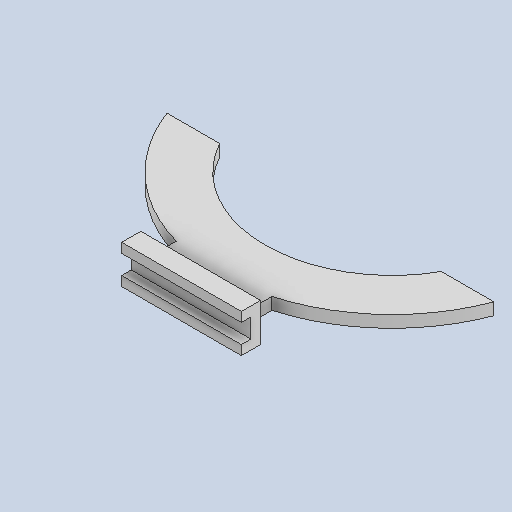
# Autodesk Inventor part: BigHolder
Saved by Autodesk Inventor 2025 (Build 290162000, 162)
## iProperties
Created: 2025-08-07
Part Number: BigHolder
Material: Generic
Document SubType Name: Modeling
Designer: Pravoslav
Density: 1 g/cm^3
Appearance: Default
Author: Pravoslav
Autodesk Inventor part; units mm, degrees
ref_plane "YZ Plane" through (0, 0, 0) normal (1, 0, 0) x (0, 1, 0)
ref_plane "XZ Plane" through (0, 0, 0) normal (0, 1, 0) x (-1, 0, 0)
ref_plane "XY Plane" through (0, 0, 0) normal (0, 0, 1) x (1, 0, 0)
sketch "Sketch1" plane through (0, 0, 0) normal (0, 1, 0) x (-1, 0, 0)
  circle A0 centre (0, 0) radius 26.5
  circle A1 centre (0, 0) radius 36.5
  line L0 (10, 40) -> (-10, 40)
  line L1 (-10, 40) -> (-10, 33)
  line L2 (-10, 33) -> (10, 33)
  line L3 (10, 33) -> (10, 40)
  line L4 (10, 40) -> (-10, 33) construction
  line L5 (-10, 40) -> (10, 33) construction
  line L6 (34.1488, 12.8883) -> (-34.1488, 12.8883)
  point P0 (0, 36.5)
  point P1 (-10, 35.1034)
  point P2 (-23.1547, 12.8883)
  point P3 (23.1547, 12.8883)
  point P4 (10, 35.1034)
  dimension "d0" = 53
  dimension "d1" = 10
  dimension "d2" = 20
  dimension "d3" = 7
  constraints: 14 end point, 3 point on circle, 2 centre point, 2 coincident, 2 horizontal, 2 midpoint, 2 parallel, 1 perpendicular
  measures "d0" diameter of A0
  measures "d1" radial gap between concentric circles of A1 A0
  measures "d2" distance of L2.end L1.end
  measures "d3" distance of L1.end L0.end
extrude "Extrusion1" add sketch "Sketch1" along normal blind 2.5 contours A0 L6 A1 L1 L2 L3 | L3 L2 L1 A1 | A1 L1 L0 L3
sketch "Sketch3" plane through (-10, 0, 40) normal (0, 0, 1) x (1, 0, 0)
  line L0 (-2.5, 5.5) -> (22.5, 5.5)
  line L1 (22.5, 5.5) -> (22.5, -2.5)
  line L2 (22.5, -2.5) -> (-2.5, -2.5)
  line L3 (-2.5, -2.5) -> (-2.5, 5.5)
  line L4 (0, 2.5) -> (20, 2.5) projected
  line L5 (0, 0) -> (0, 2.5) projected
  point P0 (10, 0)
  dimension "d6" = 25
  dimension "d7" = 8
  dimension "d8" = 3
  dimension "d9" = 2.5
  constraints: 8 end point, 2 parallel, 1 horizontal, 1 perpendicular
  measures "d6" distance of L1.end L2.end
  measures "d7" distance of L0.end L1.end
  measures "d8" distance between parallel lines of L4 L0
  measures "d9" distance between parallel lines of L3 L5
extrude "Extrusion2" add sketch "Sketch3" along normal blind 2
sketch "Sketch4" plane through (-10, 0, 42) normal (0, 0, 1) x (1, 0, 0)
  line L0 (-2.5, 5.5) -> (-2.5, -2.5) projected
  line L1 (22.5, -2.5) -> (22.5, 5.5) projected
  line L2 (-2.5, 5.5) -> (22.5, 5.5)
  line L3 (22.5, 5.5) -> (22.5, 3.5)
  line L4 (22.5, 3.5) -> (-2.5, 3.5)
  line L5 (-2.5, 3.5) -> (-2.5, 5.5)
  line L6 (-2.5, -2.5) -> (22.5, -2.5) projected
  line L7 (-2.5, -2.5) -> (22.5, -2.5)
  line L8 (22.5, -2.5) -> (22.5, -0.5)
  line L9 (22.5, -0.5) -> (-2.5, -0.5)
  line L10 (-2.5, -0.5) -> (-2.5, -2.5)
  point P0 (10, 0)
  point P1 (-2.5, -0.5)
  dimension "d12" = 2
  dimension "d13" = 2
  constraints: 16 end point, 4 parallel, 2 horizontal, 2 perpendicular, 2 point on line
  measures "d12" distance of L2.end L3.end
  measures "d13" distance of L8.end L7.end
extrude "Extrusion3" add sketch "Sketch4" along normal blind 2 contours L2 L1 L4 L0 | L9 L1 L6 L0
body "Solid1"
